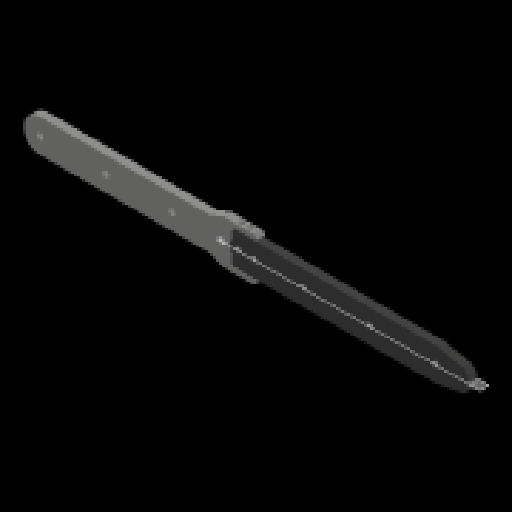
# Autodesk Inventor part: OuterDrive3DP
Saved by Autodesk Inventor 2024.1 (Build 281209000, 209)
## iProperties
Created: 2025-06-20
Part Number: OuterDrive3DP
Material: Generic
Document SubType Name: Modeling
Designer: Teddy
Density: 1 g/cm^3
Appearance: Default
Author: Teddy
Autodesk Inventor part; units mm, degrees
ref_plane "YZ Plane" through (0, 0, 0) normal (1, 0, 0) x (0, 1, 0)
ref_plane "XZ Plane" through (0, 0, 0) normal (0, 1, 0) x (-1, 0, 0)
ref_plane "XY Plane" through (0, 0, 0) normal (0, 0, 1) x (1, 0, 0)
sketch "Sketch1" plane through (0, 0, 0) normal (0, 0, 1) x (1, 0, 0)
  circle A0 centre (0, 0) radius 2.032 projected
  circle A1 centre (0, 0) radius 2.54
  line L0 (0, 0) -> (25.4, 0) construction
  line L1 (25.4, 0) -> (25.4, 7.62)
  line L2 (25.4, 7.62) -> (0, 12.7)
  circle A2 centre (-50.8, 0) radius 2.54
  circle A3 centre (-101.6, 0) radius 2.54
  circle A4 centre (-152.4, 0) radius 2.54
  circle A5 centre (-203.2, 0) radius 2.54
  circle A6 centre (-254, 0) radius 2.54
  circle A7 centre (-304.8, 0) radius 2.54
  circle A8 centre (-152.4, 0) radius 6.35
  circle A9 centre (-165.1, 0) radius 2.54
  circle A10 centre (-139.7, 0) radius 2.54
  line L3 (0, 12.7) -> (-152.4, 12.7)
  line L4 (-152.4, 12.7) -> (-152.4, 0) construction
  line L5 (25.4, 0) -> (25.4, -7.62)
  line L6 (25.4, -7.62) -> (0, -12.7)
  line L7 (0, -12.7) -> (-152.4, -12.7)
  line L8 (-152.4, 12.7) -> (-156.21, 12.7)
  line L9 (-156.21, 12.7) -> (-156.21, 5.08)
  line L10 (-152.4, -12.7) -> (-156.21, -12.7)
  line L11 (-156.21, -12.7) -> (-156.21, -5.08)
  dimension "d0" = 5.08
  dimension "d2" = 25.4
  dimension "d4" = 12.7
  dimension "d5" = 7.62
  dimension "d8" = 50.8
  dimension "d13" = 12.7
  dimension "d14" = 5.08
  dimension "d15" = 5.08
  dimension "d16" = 12.7
  dimension "d17" = 12.7
  dimension "d18" = 7.62
  dimension "d19" = 12.7
  dimension "d20" = 3.81
  constraints: 24 end point, 10 centre point, 6 horizontal, 3 vertical, 3 vertical alignment, 2 coincident, 2 horizontal alignment, 2 perpendicular, 2 point on circle, 12 other
  measures "d0" diameter of A1
  measures "d2" distance of L0.start L0.end
  measures "d4" distance of point (0, 0) L2.end
  measures "d5" distance of L0.end L1.end
  measures "d8" distance of L0.start A2.centre
  measures "d13" diameter of A8
  measures "d14" diameter of A9
  measures "d15" diameter of A10
  measures "d16" distance of A4.centre A9.centre
  measures "d17" distance of A10.centre A4.centre
  measures "d18" distance of L0.end L5.end
  measures "d19" distance from line of L0 L6.end
  measures "d20" distance of L3.end L8.end
extrude "Extrusion1" add sketch "Sketch1" along normal blind 6.35 contours L5 L6 L7 L10 L11 A8 L9 L8 L3 L2 L1 | A8
fillet "Fillet1" radius 6.35 4 edges at (0, 12.7, 3.175) (25.4, 7.62, 3.175) (25.4, -7.62, 3.175) (0, -12.7, 3.175)
sketch "Sketch2" plane through (-156.21, 12.7, 6.35) normal (0, 1, 0) x (1, 0, 0)
  circle A0 centre (3.81, 3.175) radius 2.286
  line L0 (0, 6.35) -> (0, 0) projected
  circle A1 centre (10.16, 3.175) radius 2.286
  point P0 (156.21, 6.35)
  point P1 (0, 3.175)
  dimension "d24" = 4.572
  dimension "d25" = 3.81
  dimension "d28" = 4.572
  dimension "d29" = 6.35
  constraints: 2 centre point, 2 horizontal alignment, 1 midpoint
  measures "d24" diameter of A0
  measures "d25" distance from line of L0 A0.centre
  measures "d28" diameter of A1
  measures "d29" distance of A0.centre A1.centre
extrude "Extrusion2" cut sketch "Sketch2" against normal blind 3.81
ref_plane "Work Plane1" through (-156.21, 0, 6.35) normal (0, 1, 0) x (1, 0, 0)
mirror "Mirror1" about plane through (-156.21, 0, 6.35) normal (0, 1, 0) of "Extrusion2"
fillet "Fillet2" radius 1.27 2 edges at (-156.21, 12.7, 3.175) (-156.21, -12.7, 3.175)
fillet "Fillet3" radius 1.27 2 edges at (-156.21, 5.08, 3.175) (-156.21, -5.08, 3.175)
sketch "Sketch3" plane through (0, 0, 6.35) normal (0, 0, 1) x (1, 0, 0)
  arc A0 (-156.21, -11.43) -> (-154.94, -12.7) centre (-154.94, -11.43) ccw projected
  line L0 (-154.94, -12.7) -> (-0.6288, -12.7) projected
  arc A1 (-0.6288, -12.7) -> (0.6166, -12.5767) centre (-0.6288, -6.35) ccw projected
  line L1 (0.6166, -12.5767) -> (20.2953, -8.6409) projected
  arc A2 (20.2953, -8.6409) -> (25.4, -2.4142) centre (19.05, -2.4142) ccw projected
  line L2 (25.4, -2.4142) -> (25.4, 2.4142) projected
  arc A3 (25.4, 2.4142) -> (20.2953, 8.6409) centre (19.05, 2.4142) ccw projected
  line L3 (20.2953, 8.6409) -> (0.6166, 12.5767) projected
  arc A4 (0.6166, 12.5767) -> (-0.6288, 12.7) centre (-0.6288, 6.35) ccw projected
  line L4 (-0.6288, 12.7) -> (-154.94, 12.7) projected
  arc A5 (-154.94, 12.7) -> (-156.21, 11.43) centre (-154.94, 11.43) ccw projected
  line L5 (-156.21, 11.43) -> (-156.21, 5.6796) projected
  arc A6 (-156.6333, 4.733) -> (-156.21, 5.6796) centre (-157.48, 5.6796) ccw projected
  arc A7 (-156.6333, 4.733) -> (-156.6333, -4.733) centre (-152.4, 0) ccw projected
  arc A8 (-156.21, -5.6796) -> (-156.6333, -4.733) centre (-157.48, -5.6796) ccw projected
  line L6 (-156.21, -5.6796) -> (-156.21, -11.43) projected
  circle A9 centre (-139.7, 0) radius 2.54 projected
  circle A10 centre (-101.6, 0) radius 2.54 projected
  circle A11 centre (-50.8, 0) radius 2.54 projected
  circle A12 centre (0, 0) radius 2.54 projected
  line L7 (-156.6547, 5.6796) -> (-156.6547, 11.43)
  arc A13 (-154.94, 13.1447) -> (-156.6547, 11.43) centre (-154.94, 11.43) ccw
  arc A14 (-156.6547, -11.43) -> (-154.94, -13.1447) centre (-154.94, -11.43) ccw
  line L8 (-156.6547, -11.43) -> (-156.6547, -5.6796)
  arc A15 (-156.6547, -5.6796) -> (-156.9298, -5.0645) centre (-157.48, -5.6796) ccw
  arc A16 (-156.9298, 5.0645) -> (-156.9298, -5.0645) centre (-152.4, 0) ccw
  arc A17 (-156.9298, 5.0645) -> (-156.6547, 5.6796) centre (-157.48, 5.6796) ccw
  line L9 (-154.94, 13.1447) -> (-137.16, 13.1447)
  line L10 (-137.16, 13.1447) -> (-137.16, 14.4147)
  line L11 (-137.16, 14.4147) -> (-139.7, 16.9547)
  line L12 (-139.7, 16.9547) -> (-164.2747, 16.9547)
  line L13 (-152.4, 0) -> (-139.7, 0) construction
  line L14 (-154.94, -13.1447) -> (-137.16, -13.1447)
  line L15 (-137.16, -13.1447) -> (-137.16, -14.4147)
  line L16 (-137.16, -14.4147) -> (-139.7, -16.9547)
  line L17 (-139.7, -16.9547) -> (-164.2747, -16.9547)
  line L18 (-164.2747, -16.9547) -> (-173.1647, -12.7)
  line L19 (-164.2747, 16.9547) -> (-173.1647, 12.7)
  line L20 (-173.1647, 12.7) -> (-304.8, 12.7)
  circle A18 centre (-101.6, 0) radius 2.54 construction
  circle A19 centre (-152.4, 0) radius 2.54 construction
  circle A20 centre (-203.2, 0) radius 2.54
  circle A21 centre (-254, 0) radius 2.54
  circle A22 centre (-304.8, 0) radius 2.54
  line L21 (-173.1647, -12.7) -> (-304.8, -12.7)
  arc A23 (-304.8, 12.7) -> (-304.8, -12.7) centre (-304.8, 0) ccw
  circle A24 centre (-165.1, 0) radius 2.54
  dimension "d32" = 17.78
  dimension "d33" = 1.27
  dimension "d34" = 3.81
  dimension "d35" = 45
  dimension "d36" = 7.62
  dimension "d37" = 8.89
  dimension "d40" = 50.8
  dimension "d51" = 5.08
  dimension "d52" = 12.7
  constraints: 30 end point, 12 centre point, 12 point on circle, 7 horizontal, 4 symmetric about line, 2 horizontal alignment, 2 tangent, 2 vertical, 2 vertical alignment, 1 coincident, 1 perpendicular, 1 point on line, 14 other
  measures "d32" distance of L9.start L9.end
  measures "d33" distance of L9.end L10.end
  measures "d34" distance between parallel lines of L9 L12
  measures "d35" angle of L11 L10
  measures "d36" distance from line of L7 L12.end
  measures "d37" horizontal distance of L17.end L18.end
  measures "d40" distance of A18.centre A19.centre
  measures "d51" diameter of A24
  measures "d52" distance of L13.start A24.centre
extrude "Extrusion3" add sketch "Sketch3" against normal up to surface (6.35 mm away) separate body contours A17 A16 A15 L8 A14 L14 L15 L16 L17 L18 L21 A23 L20 L19 L12 L11 L10 L9 A13 L7
sketch "Sketch4" plane through (-164.2747, 16.9547, 6.35) normal (0, 1, 0) x (1, 0, 0)
  circle A0 centre (11.8747, 3.175) radius 2.286 projected
  circle A1 centre (18.2247, 3.175) radius 2.286 projected
  circle A2 centre (18.2247, 3.175) radius 2.286 projected
  point P0 (164.2747, 6.35)
extrude "Extrusion4" cut sketch "Sketch4" against normal through all bodies 2
fillet "Fillet4" radius 1.27 4 edges at (-137.16, -13.1447, 3.175) (-137.16, -14.4147, 3.175) (-137.16, 14.4147, 3.175) (-137.16, 13.1447, 3.175)
fillet "Fillet5" radius 5.08 6 edges at (-139.7, 16.9547, 3.175) (-139.7, -16.9547, 3.175) (-164.2747, -16.9547, 3.175) (-173.1647, -12.7, 3.175) (-173.1647, 12.7, 3.175) (-164.2747, 16.9547, 3.175)
body "Solid1"
